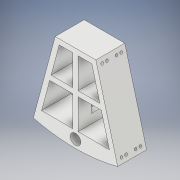
# Autodesk Inventor part: CA001
Saved by Autodesk Inventor 2017 SP1 (Build 210196100, 196)
## iProperties
Created: 2017-06-04
Part Number: CA001
Material: ABS Plastic
Document SubType Name: Modeling
Designer: Zach
Density: 1.06 g/cm^3
Appearance: CR White
Author: Zach
Autodesk Inventor part; units mm, degrees
ref_plane "YZ Plane" through (0, 0, 0) normal (1, 0, 0) x (0, 1, 0)
ref_plane "XZ Plane" through (0, 0, 0) normal (0, 1, 0) x (-1, 0, 0)
ref_plane "XY Plane" through (0, 0, 0) normal (0, 0, 1) x (1, 0, 0)
sketch "Sketch1" plane through (0, 0, 0) normal (0, 0, 1) x (1, 0, 0)
  line L0 (0, 0) -> (160, 0)
  line L1 (160, 0) -> (118.589, 154.5481)
  line L2 (41.411, 154.5481) -> (0, 0)
  line L3 (41.411, 154.5481) -> (118.589, 154.5481)
  dimension "d0" = 160
  dimension "d1" = 160
  dimension "d2" = 75
  dimension "d8" = 75
  constraints: 8 end point, 2 horizontal
  measures "d0" distance of L0.start L0.end
  measures "d1" distance of L1.end L0.end
  measures "d2" angle of L1 L0
  measures "d8" angle of L0 L2
extrude "Extrusion1" add sketch "Sketch1" along normal blind 55
sketch "Sketch7" plane through (0, 0, 0) normal (0, 0, -1) x (-1, 0, 0)
  circle A0 centre (-80, 304.672) radius 315 construction
  line L0 (0, 0) -> (-160, 0) projected
  arc A1 (-160, 0) -> (0, 0) centre (-80, 304.672) ccw
  dimension "d28" = 630
  constraints: 4 point on circle, 2 centre point, 1 concentric
  measures "d28" diameter of A0
extrude "Extrusion6" add sketch "Sketch7" against normal blind 55
sketch "Sketch19" plane through (0, 0, 0) normal (0, 0, -1) x (-1, 0, 0)
  circle A0 centre (-80, 4.836) radius 10
  line L0 (-118.589, 154.5481) -> (-41.411, 154.5481) projected
  line L1 (-80, 154.5481) -> (-80, -10.328)
  arc A1 (-160, 0) -> (0, 0) centre (-80, 304.672) ccw projected
  dimension "d112" = 20
  dimension "d113" = 15.164
  constraints: 2 end point, 1 centre point, 1 midpoint, 1 point on circle, 1 point on line, 1 vertical
  measures "d112" diameter of A0
  measures "d113" distance of L1.end A0.centre
extrude "Extrusion19" cut sketch "Sketch19" against normal through all
sketch "Sketch20" plane through (0, 0, 0) normal (0, 0, -1) x (-1, 0, 0)
  line L0 (-41.411, 154.5481) -> (0, 0) projected
  circle A0 centre (-80, 4.836) radius 10 projected
  line L1 (-41.411, 154.5481) -> (0, 0) projected
  line L2 (-118.589, 154.5481) -> (-41.411, 154.5481) projected
  line L3 (-160, 0) -> (-118.589, 154.5481) projected
  arc A1 (-160, 0) -> (0, 0) centre (-80, 304.672) ccw projected
  line L4 (-49.0843, 144.5481) -> (-12.3033, 7.2797)
  arc A2 (-147.6967, 7.2797) -> (-12.3033, 7.2797) centre (-80, 304.672) ccw
  line L5 (-147.6967, 7.2797) -> (-110.9157, 144.5481)
  line L6 (-110.9157, 144.5481) -> (-49.0843, 144.5481)
  line L7 (-15.6678, 19.836) -> (-144.3322, 19.836)
  dimension "d116" = 10
  dimension "d119" = 15
  constraints: 8 end point, 2 point on circle, 2 point on line, 1 centre point, 1 horizontal, 3 other
  measures "d116" distance between parallel lines of L2 L6
  measures "d119" distance from line of L7 A0.centre
extrude "Extrusion20" cut sketch "Sketch20" against normal through all contours L5 L6 L4 L7
sketch "Sketch21" plane through (0, 0, 0) normal (0, 0, -1) x (-1, 0, 0)
  line L0 (-110.9157, 144.5481) -> (-49.0843, 144.5481) projected
  line L1 (-75, 144.5481) -> (-75, 19.836)
  line L2 (-15.6678, 19.836) -> (-144.3322, 19.836) projected
  line L3 (-85, 19.836) -> (-85, 144.5481)
  line L4 (-85, 144.5481) -> (-75, 144.5481)
  line L5 (-75, 19.836) -> (-85, 19.836)
  point P0 (0, 0)
  point P1 (-80, 144.5481)
  point P2 (-80, 144.5481)
  dimension "d120" = 10
  constraints: 8 end point, 3 point on line, 2 midpoint, 2 perpendicular, 1 coincident, 1 parallel, 1 vertical
  measures "d120" distance between parallel lines of L3 L1
extrude "Extrusion21" add sketch "Sketch21" against normal blind 55
sketch "Sketch22" plane through (0, 0, 0) normal (0, 0, -1) x (-1, 0, 0)
  line L0 (-15.6678, 19.836) -> (-49.0843, 144.5481) projected
  line L1 (-33.7158, 87.1921) -> (-126.2842, 87.1921)
  line L2 (-110.9157, 144.5481) -> (-144.3322, 19.836) projected
  line L3 (-80, 87.1921) -> (-80, 77.1921)
  line L4 (-31.0363, 77.1921) -> (-128.9637, 77.1921)
  line L5 (-75, 19.836) -> (-75, 144.5481) projected
  line L6 (-33.7158, 87.1921) -> (-31.0363, 77.1921)
  line L7 (-126.2842, 87.1921) -> (-128.9637, 77.1921)
  point P0 (0, 0)
  point P1 (-80, 82.1921)
  point P2 (-75, 82.1921)
  dimension "d124" = 10
  constraints: 10 end point, 4 midpoint, 4 point on line, 2 collinear, 2 horizontal, 1 horizontal alignment
  measures "d124" distance between parallel lines of L4 L1
extrude "Extrusion22" add sketch "Sketch22" against normal blind 55
sketch "Sketch23" plane through (0, 0, 0) normal (0, 0, -1) x (-1, 0, 0)
  circle A0 centre (-80, 60) radius 55
  line L0 (-118.589, 154.5481) -> (-41.411, 154.5481) projected
  line L1 (-57.5, 82.5) -> (-102.5, 82.5)
  line L2 (-102.5, 82.5) -> (-102.5, 37.5)
  line L3 (-102.5, 37.5) -> (-57.5, 37.5)
  line L4 (-57.5, 37.5) -> (-57.5, 82.5)
  point P0 (0, 0)
  point P1 (-80, 154.5481)
  point P2 (-102.5, 60)
  point P3 (-80, 82.5)
  dimension "d127" = 110
  dimension "d128" = 60
  dimension "d129" = 45
  dimension "d130" = 45
  constraints: 8 end point, 3 midpoint, 2 parallel, 2 vertical alignment, 1 centre point, 1 horizontal, 1 horizontal alignment, 1 perpendicular
  measures "d127" diameter of A0
  measures "d128" vertical distance of point (0, 0) A0.centre
  measures "d129" distance of L3.end L2.end
  measures "d130" distance of L2.end L1.end
extrude "Extrusion23" cut sketch "Sketch23" against normal blind 30 contours L4 L3 L2 L1
sketch "Sketch24" plane through (118.589, 154.5481, 55) normal (0.9659, 0.2588, 0) x (0, 0, -1)
  line L0 (45.475, -9.525) -> (45.475, -150.475) construction
  line L1 (9.525, -150.475) -> (9.525, -9.525) construction
  line L2 (0, -160) -> (0, 0) construction
  circle A0 centre (45.475, -150.475) radius 2.5
  circle A1 centre (9.525, -150.475) radius 2.5
  circle A2 centre (9.525, -9.525) radius 2.5
  circle A3 centre (45.475, -9.525) radius 2.5
  circle A4 centre (18.4199, -150.475) radius 2.5
  circle A5 centre (36.5801, -150.475) radius 2.5
  circle A6 centre (36.5801, -9.525) radius 2.5
  circle A7 centre (18.4199, -9.525) radius 2.5
  point P0 (55, -118.589)
  point P1 (9.525, -80)
  point P2 (0, -80)
  dimension "d133" = 140.95
  dimension "d134" = 140.95
  dimension "d135" = 9.525
  dimension "d136" = 9.525
  dimension "d137" = 5
  dimension "d138" = 5
  dimension "d139" = 5
  dimension "d140" = 5
  dimension "d141" = 5
  dimension "d142" = 5
  dimension "d143" = 5
  dimension "d144" = 5
  dimension "d145" = 18.4199
  dimension "d146" = 18.4199
  constraints: 8 centre point, 6 horizontal alignment, 4 coincident, 4 end point, 2 midpoint, 2 vertical, 2 vertical alignment
  measures "d133" distance of L0.start L0.end
  measures "d134" distance of L1.start L1.end
  measures "d135" distance from line of point (55, -118.589) L0
  measures "d136" distance between parallel lines of L2 L1
  measures "d137" diameter of A0
  measures "d138" diameter of A1
  measures "d139" diameter of A2
  measures "d140" diameter of A3
  measures "d141" diameter of A4
  measures "d142" diameter of A5
  measures "d143" diameter of A6
  measures "d144" diameter of A7
  measures "d145" distance from line of L2 A4.centre
  measures "d146" horizontal distance of point (55, -118.589) A5.centre
extrude "Extrusion24" cut sketch "Sketch24" against normal blind 25
sketch "Sketch25" plane through (41.411, 154.5481, 0) normal (-0.9659, 0.2588, 0) x (0, 0, 1)
  line L0 (45.475, -9.525) -> (45.475, -150.475) construction
  line L1 (9.525, -150.475) -> (9.525, -9.525) construction
  circle A0 centre (45.475, -150.475) radius 2.5
  circle A1 centre (9.525, -150.475) radius 2.5
  circle A2 centre (9.525, -9.525) radius 2.5
  circle A3 centre (45.475, -9.525) radius 2.5
  circle A4 centre (18.4199, -150.475) radius 2.5
  circle A5 centre (36.5801, -150.475) radius 2.5
  circle A6 centre (36.5801, -9.525) radius 2.5
  circle A7 centre (18.4199, -9.525) radius 2.5
  line L2 (0, 0) -> (0, -160) projected
  line L3 (55, 0) -> (55, -160) projected
  point P0 (9.525, -80)
  point P1 (0, -80)
  dimension "d149" = 140.95
  dimension "d150" = 140.95
  dimension "d153" = 5
  dimension "d154" = 5
  dimension "d155" = 5
  dimension "d156" = 5
  dimension "d157" = 5
  dimension "d158" = 5
  dimension "d159" = 5
  dimension "d160" = 5
  dimension "d163" = 9.525
  dimension "d164" = 18.4199
  dimension "d165" = 18.4199
  dimension "d166" = 9.525
  constraints: 8 centre point, 6 horizontal alignment, 4 coincident, 4 end point, 2 midpoint, 2 vertical, 2 vertical alignment
  measures "d149" distance of L0.start L0.end
  measures "d150" distance of L1.start L1.end
  measures "d153" diameter of A0
  measures "d154" diameter of A1
  measures "d155" diameter of A2
  measures "d156" diameter of A3
  measures "d157" diameter of A4
  measures "d158" diameter of A5
  measures "d159" diameter of A6
  measures "d160" diameter of A7
  measures "d163" distance from line of L2 L1.end
  measures "d164" distance from line of L2 A7.centre
  measures "d165" distance from line of L3 A6.centre
  measures "d166" distance from line of L3 A3.centre
extrude "Extrusion25" cut sketch "Sketch25" against normal blind 25
body "Solid1"
